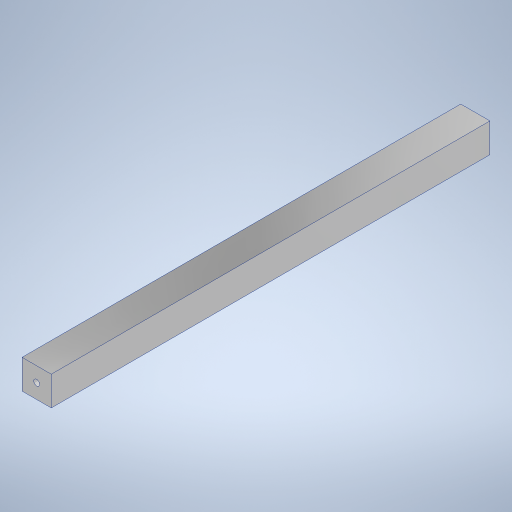
# Autodesk Inventor part: 2020x260mm
Saved by Autodesk Inventor 2024 (Build 280153000, 153)
## iProperties
Created: 2023-08-11
Part Number: 2020x260mm
Material: ABS Plastic
Document SubType Name: Modeling
Designer: l1534
Density: 1.06 g/cm^3
Appearance: Aluminum - Flat
Author: l1534
Autodesk Inventor part; units mm, degrees
ref_plane "YZ Plane" through (0, 0, 0) normal (1, 0, 0) x (0, 1, 0)
ref_plane "XZ Plane" through (0, 0, 0) normal (0, 1, 0) x (-1, 0, 0)
ref_plane "XY Plane" through (0, 0, 0) normal (0, 0, 1) x (1, 0, 0)
sketch "Sketch1" plane through (0, 0, 0) normal (0, 0, 1) x (1, 0, 0)
  line L0 (-11.9064, 7.7279) -> (8.0936, 7.7279)
  line L1 (8.0936, 7.7279) -> (8.0936, -12.2721)
  line L2 (8.0936, -12.2721) -> (-11.9064, -12.2721)
  line L3 (-11.9064, -12.2721) -> (-11.9064, 7.7279)
  point P0 (0, 0)
  dimension "d0" = 20
  dimension "d1" = 20
  constraints: 8 end point, 2 parallel, 1 horizontal, 1 perpendicular
  measures "d0" distance of L0.start L0.end
  measures "d1" distance of L0.end L1.end
extrude "Extrusion1" add sketch "Sketch1" along normal blind 300
sketch "Sketch2" plane through (0, 0, 300) normal (0, 0, 1) x (1, 0, 0)
  circle A0 centre (-1.9064, -2.2721) radius 2
  line L0 (-11.9064, -12.2721) -> (8.0936, -12.2721) projected
  line L1 (8.0936, -12.2721) -> (8.0936, 7.7279) projected
  point P0 (0, 0)
  dimension "d4" = 4
  dimension "d5" = 10
  dimension "d6" = 10
  constraints: 1 centre point
  measures "d4" diameter of A0
  measures "d5" distance from line of L0 A0.centre
  measures "d6" distance from line of L1 A0.centre
extrude "Extrusion2" cut sketch "Sketch2" against normal blind 250
body "Solid1"
